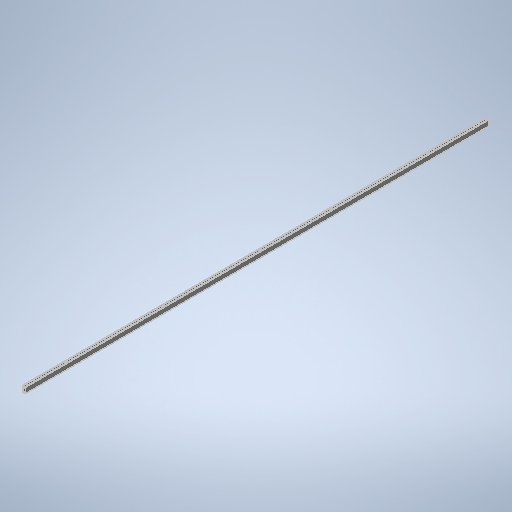
# Autodesk Inventor part: SP40-11 JUNTA DE FELPA PARA ENCUENTRO HOJA CORREDERA 695 mm
Saved by Autodesk Inventor 2025 (Build 290162000, 162)
## iProperties
Created: 2026-02-24
Part Number: SP40-11 JUNTA DE FELPA PARA ENCUENTRO HOJA CORREDERA 695 mm
Material: Caucho
Document SubType Name: Modeling
Designer: Frank
Density: 0.93 g/cm^3
Appearance: Gris
Author: Frank
Autodesk Inventor part; units mm, degrees
ref_plane "YZ Plane" through (0, 0, 0) normal (1, 0, 0) x (0, 1, 0)
ref_plane "XZ Plane" through (0, 0, 0) normal (0, 1, 0) x (-1, 0, 0)
ref_plane "XY Plane" through (0, 0, 0) normal (0, 0, 1) x (1, 0, 0)
sketch "Boceto1" plane through (0, 0, 0) normal (0, 0, 1) x (1, 0, 0)
  line L0 (-34.7702, -0.3498) -> (-34.7702, 2.9502)
  line L1 (-34.7702, 2.9502) -> (-33.4702, 2.9502)
  line L2 (-33.4702, 2.9502) -> (-33.4702, 0.9502)
  line L3 (-33.4702, 0.9502) -> (-32.1702, 0.9502)
  line L4 (-32.1702, 0.9502) -> (-32.1702, 8.9502)
  line L5 (-32.1702, 8.9502) -> (-33.4702, 8.9502)
  line L6 (-33.4702, 8.9502) -> (-33.4702, 6.9502)
  line L7 (-33.4702, 6.9502) -> (-34.7702, 6.9502)
  line L8 (-34.7702, 6.9502) -> (-34.7702, 10.2502)
  line L9 (-34.7702, 10.2502) -> (-35.7702, 10.2502)
  line L10 (-35.7702, 10.2502) -> (-35.7702, -0.3498)
  line L11 (-35.7702, -0.3498) -> (-34.7702, -0.3498)
  dimension "d14" = 1.3
  dimension "d41" = 1
  dimension "d42" = 4
  dimension "d43" = 10.6
  dimension "d44" = 8
  dimension "d45" = 1.3
  constraints: 24 end point, 7 perpendicular, 4 point on line, 1 horizontal
  measures "d14" distance between parallel lines of L4 L6
  measures "d41" distance of L8.end L9.end
  measures "d42" distance between parallel lines of L1 L7
  measures "d43" distance of L9.end L10.end
  measures "d44" distance of L3.end L4.end
  measures "d45" distance between parallel lines of L0 L2
extrude "Extrusión1" add sketch "Boceto1" against normal blind 695
